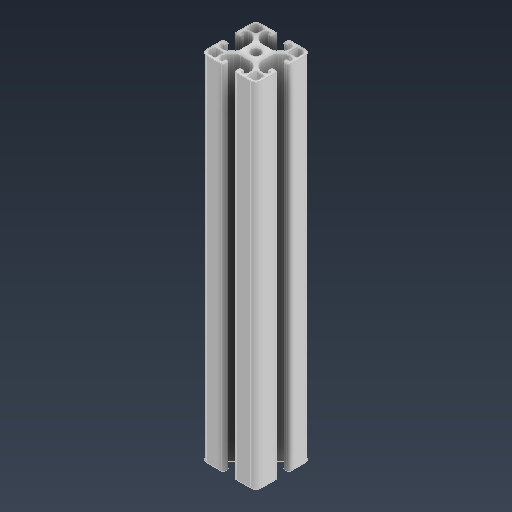
# Autodesk Inventor part: centerAxleSupportBeam
Saved by Autodesk Inventor 2021.4 (Build 254397000, 397)
## iProperties
Created: 2022-03-01
Part Number: centerAxleSupportBeam
Material: Generic
Document SubType Name: Modeling
Designer: jo_ki
Density: 1 g/cm^3
Appearance: Default
Author: jo_ki
Autodesk Inventor part; units mm, degrees
ref_plane "YZ Plane" through (0, 0, 0) normal (1, 0, 0) x (0, 1, 0)
ref_plane "XZ Plane" through (0, 0, 0) normal (0, 1, 0) x (-1, 0, 0)
ref_plane "XY Plane" through (0, 0, 0) normal (0, 0, 1) x (1, 0, 0)
derived "Profil_8_40x40_leicht.ipt"
sketch "Sketch7" plane through (0, 0, 0) normal (0, 1, 0) x (-1, 0, 0)
  arc A0 (12.3, 18.2) -> (11.8, 17.7) centre (12.3, 17.7) ccw
  line L0 (11.8, 17.7) -> (11.8, 12.3)
  arc A1 (11.8, 12.3) -> (12.3, 11.8) centre (12.3, 12.3) ccw
  line L1 (12.3, 11.8) -> (17.7, 11.8)
  arc A2 (17.7, 11.8) -> (18.2, 12.3) centre (17.7, 12.3) ccw
  line L2 (18.2, 12.3) -> (18.2, 16)
  arc A3 (18.2, 16) -> (16, 18.2) centre (16, 16) ccw
  line L3 (16, 18.2) -> (12.3, 18.2)
  arc A4 (-18.2, 12.3) -> (-17.7, 11.8) centre (-17.7, 12.3) ccw
  line L4 (-17.7, 11.8) -> (-12.3, 11.8)
  arc A5 (-12.3, 11.8) -> (-11.8, 12.3) centre (-12.3, 12.3) ccw
  line L5 (-11.8, 12.3) -> (-11.8, 17.7)
  arc A6 (-11.8, 17.7) -> (-12.3, 18.2) centre (-12.3, 17.7) ccw
  line L6 (-12.3, 18.2) -> (-16, 18.2)
  arc A7 (-16, 18.2) -> (-18.2, 16) centre (-16, 16) ccw
  line L7 (-18.2, 16) -> (-18.2, 12.3)
  arc A8 (-12.3, -18.2) -> (-11.8, -17.7) centre (-12.3, -17.7) ccw
  line L8 (-11.8, -17.7) -> (-11.8, -12.3)
  arc A9 (-11.8, -12.3) -> (-12.3, -11.8) centre (-12.3, -12.3) ccw
  line L9 (-12.3, -11.8) -> (-17.7, -11.8)
  arc A10 (-17.7, -11.8) -> (-18.2, -12.3) centre (-17.7, -12.3) ccw
  line L10 (-18.2, -12.3) -> (-18.2, -16)
  arc A11 (-18.2, -16) -> (-16, -18.2) centre (-16, -16) ccw
  line L11 (-16, -18.2) -> (-12.3, -18.2)
  arc A12 (18.2, -12.3) -> (17.7, -11.8) centre (17.7, -12.3) ccw
  line L12 (17.7, -11.8) -> (12.3, -11.8)
  arc A13 (12.3, -11.8) -> (11.8, -12.3) centre (12.3, -12.3) ccw
  line L13 (11.8, -12.3) -> (11.8, -17.7)
  arc A14 (11.8, -17.7) -> (12.3, -18.2) centre (12.3, -17.7) ccw
  line L14 (12.3, -18.2) -> (16, -18.2)
  arc A15 (16, -18.2) -> (18.2, -16) centre (16, -16) ccw
  line L15 (18.2, -16) -> (18.2, -12.3)
  circle A16 centre (0, 0) radius 3.4
  arc A17 (20, -5.5) -> (18.5, -4) centre (18.5, -5.5) ccw
  line L16 (20, -16) -> (20, -5.5)
  arc A18 (16, -20) -> (20, -16) centre (16, -16) ccw
  line L17 (5.5, -20) -> (16, -20)
  arc A19 (4, -18.5) -> (5.5, -20) centre (5.5, -18.5) ccw
  line L18 (4, -18.5) -> (4, -16.5)
  arc A20 (5, -15.5) -> (4, -16.5) centre (5, -16.5) ccw
  line L19 (5, -15.5) -> (6.5, -15.5)
  arc A21 (7, -16) -> (6.5, -15.5) centre (6.5, -16) ccw
  line L20 (7, -16) -> (7, -17.55)
  arc A22 (7, -17.55) -> (7.45, -18) centre (7.45, -17.55) ccw
  line L21 (7.45, -18) -> (7.5, -18)
  arc A23 (7.5, -18) -> (10, -15.5) centre (7.5, -15.5) ccw
  line L22 (10, -15.5) -> (10, -14.1924)
  arc A24 (10, -14.1924) -> (8.5355, -10.6569) centre (5, -14.1924) ccw
  line L23 (8.5355, -10.6569) -> (7.0931, -9.2145)
  arc A25 (7.0931, -9.2145) -> (3.5576, -7.75) centre (3.5576, -12.75) ccw
  line L24 (3.5576, -7.75) -> (-3.5576, -7.75)
  arc A26 (-3.5576, -7.75) -> (-7.0931, -9.2145) centre (-3.5576, -12.75) ccw
  line L25 (-7.0931, -9.2145) -> (-8.5355, -10.6569)
  arc A27 (-8.5355, -10.6569) -> (-10, -14.1924) centre (-5, -14.1924) ccw
  line L26 (-10, -14.1924) -> (-10, -15.5)
  arc A28 (-10, -15.5) -> (-7.5, -18) centre (-7.5, -15.5) ccw
  line L27 (-7.5, -18) -> (-7.45, -18)
  arc A29 (-7.45, -18) -> (-7, -17.55) centre (-7.45, -17.55) ccw
  line L28 (-7, -17.55) -> (-7, -16)
  arc A30 (-6.5, -15.5) -> (-7, -16) centre (-6.5, -16) ccw
  line L29 (-6.5, -15.5) -> (-5, -15.5)
  arc A31 (-4, -16.5) -> (-5, -15.5) centre (-5, -16.5) ccw
  line L30 (-4, -16.5) -> (-4, -18.5)
  arc A32 (-5.5, -20) -> (-4, -18.5) centre (-5.5, -18.5) ccw
  line L31 (-16, -20) -> (-5.5, -20)
  arc A33 (-20, -16) -> (-16, -20) centre (-16, -16) ccw
  line L32 (-20, -5.5) -> (-20, -16)
  arc A34 (-18.5, -4) -> (-20, -5.5) centre (-18.5, -5.5) ccw
  line L33 (-18.5, -4) -> (-16.5, -4)
  arc A35 (-15.5, -5) -> (-16.5, -4) centre (-16.5, -5) ccw
  line L34 (-15.5, -5) -> (-15.5, -6.5)
  arc A36 (-16, -7) -> (-15.5, -6.5) centre (-16, -6.5) ccw
  line L35 (-16, -7) -> (-17.55, -7)
  arc A37 (-17.55, -7) -> (-18, -7.45) centre (-17.55, -7.45) ccw
  line L36 (-18, -7.45) -> (-18, -7.5)
  arc A38 (-18, -7.5) -> (-15.5, -10) centre (-15.5, -7.5) ccw
  line L37 (-15.5, -10) -> (-14.1924, -10)
  arc A39 (-14.1924, -10) -> (-10.6569, -8.5355) centre (-14.1924, -5) ccw
  line L38 (-10.6569, -8.5355) -> (-9.2145, -7.0931)
  arc A40 (-9.2145, -7.0931) -> (-7.75, -3.5576) centre (-12.75, -3.5576) ccw
  line L39 (-7.75, -3.5576) -> (-7.75, 3.5576)
  arc A41 (-7.75, 3.5576) -> (-9.2145, 7.0931) centre (-12.75, 3.5576) ccw
  line L40 (-9.2145, 7.0931) -> (-10.6569, 8.5355)
  arc A42 (-10.6569, 8.5355) -> (-14.1924, 10) centre (-14.1924, 5) ccw
  line L41 (-14.1924, 10) -> (-15.5, 10)
  arc A43 (-15.5, 10) -> (-18, 7.5) centre (-15.5, 7.5) ccw
  line L42 (-18, 7.5) -> (-18, 7.45)
  arc A44 (-18, 7.45) -> (-17.55, 7) centre (-17.55, 7.45) ccw
  line L43 (-17.55, 7) -> (-16, 7)
  arc A45 (-15.5, 6.5) -> (-16, 7) centre (-16, 6.5) ccw
  line L44 (-15.5, 6.5) -> (-15.5, 5)
  arc A46 (-16.5, 4) -> (-15.5, 5) centre (-16.5, 5) ccw
  line L45 (-16.5, 4) -> (-18.5, 4)
  arc A47 (-20, 5.5) -> (-18.5, 4) centre (-18.5, 5.5) ccw
  line L46 (-20, 16) -> (-20, 5.5)
  arc A48 (-16, 20) -> (-20, 16) centre (-16, 16) ccw
  line L47 (-5.5, 20) -> (-16, 20)
  arc A49 (-4, 18.5) -> (-5.5, 20) centre (-5.5, 18.5) ccw
  line L48 (-4, 18.5) -> (-4, 16.5)
  arc A50 (-5, 15.5) -> (-4, 16.5) centre (-5, 16.5) ccw
  line L49 (-5, 15.5) -> (-6.5, 15.5)
  arc A51 (-7, 16) -> (-6.5, 15.5) centre (-6.5, 16) ccw
  line L50 (-7, 16) -> (-7, 17.55)
  arc A52 (-7, 17.55) -> (-7.45, 18) centre (-7.45, 17.55) ccw
  line L51 (-7.45, 18) -> (-7.5, 18)
  arc A53 (-7.5, 18) -> (-10, 15.5) centre (-7.5, 15.5) ccw
  line L52 (-10, 15.5) -> (-10, 14.1924)
  arc A54 (-10, 14.1924) -> (-8.5355, 10.6569) centre (-5, 14.1924) ccw
  line L53 (-8.5355, 10.6569) -> (-7.0931, 9.2145)
  arc A55 (-7.0931, 9.2145) -> (-3.5576, 7.75) centre (-3.5576, 12.75) ccw
  line L54 (-3.5576, 7.75) -> (3.5576, 7.75)
  arc A56 (3.5576, 7.75) -> (7.0931, 9.2145) centre (3.5576, 12.75) ccw
  line L55 (7.0931, 9.2145) -> (8.5355, 10.6569)
  arc A57 (8.5355, 10.6569) -> (10, 14.1924) centre (5, 14.1924) ccw
  line L56 (10, 14.1924) -> (10, 15.5)
  arc A58 (10, 15.5) -> (7.5, 18) centre (7.5, 15.5) ccw
  line L57 (7.5, 18) -> (7.45, 18)
  arc A59 (7.45, 18) -> (7, 17.55) centre (7.45, 17.55) ccw
  line L58 (7, 17.55) -> (7, 16)
  arc A60 (6.5, 15.5) -> (7, 16) centre (6.5, 16) ccw
  line L59 (6.5, 15.5) -> (5, 15.5)
  arc A61 (4, 16.5) -> (5, 15.5) centre (5, 16.5) ccw
  line L60 (4, 16.5) -> (4, 18.5)
  arc A62 (5.5, 20) -> (4, 18.5) centre (5.5, 18.5) ccw
  line L61 (16, 20) -> (5.5, 20)
  arc A63 (20, 16) -> (16, 20) centre (16, 16) ccw
  line L62 (20, 5.5) -> (20, 16)
  arc A64 (18.5, 4) -> (20, 5.5) centre (18.5, 5.5) ccw
  line L63 (18.5, 4) -> (16.5, 4)
  arc A65 (15.5, 5) -> (16.5, 4) centre (16.5, 5) ccw
  line L64 (15.5, 5) -> (15.5, 6.5)
  arc A66 (16, 7) -> (15.5, 6.5) centre (16, 6.5) ccw
  line L65 (16, 7) -> (17.55, 7)
  arc A67 (17.55, 7) -> (18, 7.45) centre (17.55, 7.45) ccw
  line L66 (18, 7.45) -> (18, 7.5)
  arc A68 (18, 7.5) -> (15.5, 10) centre (15.5, 7.5) ccw
  line L67 (15.5, 10) -> (14.1924, 10)
  arc A69 (14.1924, 10) -> (10.6569, 8.5355) centre (14.1924, 5) ccw
  line L68 (10.6569, 8.5355) -> (9.2145, 7.0931)
  arc A70 (9.2145, 7.0931) -> (7.75, 3.5576) centre (12.75, 3.5576) ccw
  line L69 (7.75, 3.5576) -> (7.75, -3.5576)
  arc A71 (7.75, -3.5576) -> (9.2145, -7.0931) centre (12.75, -3.5576) ccw
  line L70 (9.2145, -7.0931) -> (10.6569, -8.5355)
  arc A72 (10.6569, -8.5355) -> (14.1924, -10) centre (14.1924, -5) ccw
  line L71 (14.1924, -10) -> (15.5, -10)
  arc A73 (15.5, -10) -> (18, -7.5) centre (15.5, -7.5) ccw
  line L72 (18, -7.5) -> (18, -7.45)
  arc A74 (18, -7.45) -> (17.55, -7) centre (17.55, -7.45) ccw
  line L73 (17.55, -7) -> (16, -7)
  arc A75 (15.5, -6.5) -> (16, -7) centre (16, -6.5) ccw
  line L74 (15.5, -6.5) -> (15.5, -5)
  arc A76 (16.5, -4) -> (15.5, -5) centre (16.5, -5) ccw
  line L75 (16.5, -4) -> (18.5, -4)
derived "Mastersketch.ipt"
extrude "Extrusion1" add sketch "Sketch7" along normal blind 257.9477
equation "\"d2\" = ballInletWheel_diameter + 2 * ballInletWheel_margin"
equation "\"ballInletWheel_diameter\" = 237.947682"
equation "\"ballInletWheel_margin\" = 10"
body "Solid1"
